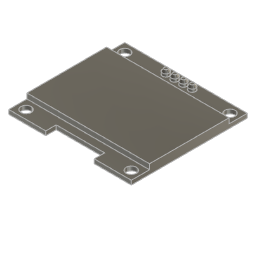
Reed Machine Case v17 (Autodesk Fusion 360 archive; units mm, degrees)
design "SSH1106+128x64+IIC+OLED+Display+1.3_+v3"
Autodesk Fusion 360 part; units mm, degrees
sketch "Sketch1" plane through (0, 0, 0) normal (0, 0, 1) x (1, 0, 0)
  line L0 (14.71, 7.35) -> (-14.71, 7.35)
  line L1 (-14.71, 7.35) -> (-14.71, -7.35)
  line L2 (-14.71, -7.35) -> (14.71, -7.35)
  line L3 (14.71, -7.35) -> (14.71, 7.35)
  line L4 (14.71, 7.35) -> (-14.71, -7.35) construction
  line L5 (-14.71, 7.35) -> (14.71, -7.35) construction
  line L6 (-17.7, 7.35) -> (-17.7, 14.7)
  line L7 (-17.7, 14.7) -> (-14.71, 14.7)
  line L8 (-17.7, 14.7) -> (17.7, 14.7)
  line L9 (17.7, 14.7) -> (17.7, -18.8)
  line L10 (17.7, -18.8) -> (-17.7, -18.8)
  line L11 (-17.7, -18.8) -> (-17.7, 14.7)
  line L12 (-17.7, 14.7) -> (6.5694, 14.7)
  line L13 (6.5694, 9.45) -> (-14.71, 9.45)
  line L14 (-17.7, 9.45) -> (-17.7, 14.7)
  line L15 (17.7, 9.45) -> (-17.7, 9.45)
  line L16 (-17.7, 9.45) -> (-17.7, -13.55)
  line L17 (-17.7, -13.55) -> (17.7, -13.55)
  line L18 (17.7, -13.55) -> (17.7, 9.45)
  line L19 (-17.7, 14.7) -> (-15.2, 14.7)
  line L20 (-15.2, 14.7) -> (-15.2, 12.2)
  line L21 (-15.2, 12.2) -> (-17.7, 12.2)
  line L22 (-17.7, 12.2) -> (-17.7, 14.7)
  circle A0 centre (-15.2, 12.2) radius 1.5
  circle A1 centre (15.2, 12.2) radius 1.5
  circle A2 centre (-15.2, -16.3) radius 1.5
  circle A3 centre (15.2, -16.3) radius 1.5
  line L23 (-17.7, -18.8) -> (-7, -18.8)
  line L24 (-7, -18.8) -> (-7, -17.6734)
  line L25 (-7, -17.6734) -> (-17.7, -17.6734)
  line L26 (-17.7, -17.6734) -> (-17.7, -18.8)
  line L27 (-7, -18.8) -> (7, -18.8)
  line L28 (7, -18.8) -> (7, -15.8)
  line L29 (7, -15.8) -> (-7, -15.8)
  line L30 (-7, -15.8) -> (-7, -18.8)
  line L31 (-17.7, 14.7) -> (-3.81, 14.7)
  line L32 (-3.81, 14.7) -> (-3.81, 12.7)
  line L33 (-3.81, 12.7) -> (-17.7, 12.7)
  line L34 (-17.7, 12.7) -> (-17.7, 14.7)
  circle A4 centre (-3.81, 12.7) radius 1
  circle A5 centre (-3.81, 12.7) radius 1
  circle A6 centre (-3.81, 12.7) radius 1
  circle A7 centre (-1.27, 12.7) radius 1
  circle A8 centre (1.27, 12.7) radius 1
  circle A9 centre (3.81, 12.7) radius 1
  circle A10 centre (-3.81, 12.7) radius 0.5
  circle A11 centre (-1.27, 12.7) radius 0.5
  circle A12 centre (1.27, 12.7) radius 0.5
  circle A13 centre (3.81, 12.7) radius 0.5
  line L35 (-2.81, 13.7) -> (-4.81, 13.7)
  line L36 (-4.81, 13.7) -> (-4.81, 11.7)
  line L37 (-4.81, 11.7) -> (-2.81, 11.7)
  line L38 (-2.81, 11.7) -> (-2.81, 13.7)
  line L39 (-2.81, 13.7) -> (-4.81, 11.7) construction
  line L40 (-4.81, 13.7) -> (-2.81, 11.7) construction
  line L41 (-0.27, 13.7) -> (-2.27, 13.7)
  line L42 (-2.27, 13.7) -> (-2.27, 11.7)
  line L43 (-2.27, 11.7) -> (-0.27, 11.7)
  line L44 (-0.27, 11.7) -> (-0.27, 13.7)
  line L45 (-0.27, 13.7) -> (-2.27, 11.7) construction
  line L46 (-2.27, 13.7) -> (-0.27, 11.7) construction
  line L47 (2.27, 13.7) -> (0.27, 13.7)
  line L48 (0.27, 13.7) -> (0.27, 11.7)
  line L49 (0.27, 11.7) -> (2.27, 11.7)
  line L50 (2.27, 11.7) -> (2.27, 13.7)
  line L51 (2.27, 13.7) -> (0.27, 11.7) construction
  line L52 (0.27, 13.7) -> (2.27, 11.7) construction
  line L53 (4.81, 13.7) -> (2.81, 13.7)
  line L54 (2.81, 13.7) -> (2.81, 11.7)
  line L55 (2.81, 11.7) -> (4.81, 11.7)
  line L56 (4.81, 11.7) -> (4.81, 13.7)
  line L57 (4.81, 13.7) -> (2.81, 11.7) construction
  line L58 (2.81, 13.7) -> (4.81, 11.7) construction
  point P0 (-3.81, 12.7)
  point P1 (-1.27, 12.7)
  point P2 (1.27, 12.7)
  point P3 (3.81, 12.7)
  dimension "d1" = 29.42
  dimension "d2" = 14.7
  dimension "d3" = 2.99
  dimension "d5" = 35.4
  dimension "d6" = 33.5
  dimension "d7" = 5.25
  dimension "d8" = 23
  dimension "d9" = 2.5
  dimension "d10" = 2.5
  dimension "d11" = 3
  dimension "d12" = 3
  dimension "d13" = 3
  dimension "d14" = 3
  dimension "d19" = 10.7
  dimension "d20" = 14
  dimension "d21" = 3
  dimension "d24" = 13.89
  dimension "d25" = 2
  dimension "d26" = 2
  dimension "d27" = 2
  dimension "d28" = 2
  dimension "d29" = 2
  dimension "d30" = 2
  dimension "d31" = 2
  dimension "d34" = 1
  dimension "d35" = 1
  dimension "d36" = 1
  dimension "d37" = 1
  dimension "d42" = 2
  dimension "d43" = 2
  dimension "d44" = 2
  dimension "d45" = 2
  dimension "d46" = 2
  dimension "d47" = 2
  dimension "d48" = 2
  dimension "d49" = 2
  constraint horizontal L0
  constraint perpendicular L0 L1
  constraint parallel L0 L2
  constraint parallel L1 L3
  constraint coincident L4 origin
  constraint coincident L5 origin
  constraint vertical L6
  constraint horizontal L7
  constraint horizontal L8
  constraint vertical L9
  constraint horizontal L10
  constraint vertical L11
  constraint horizontal L12
  constraint horizontal L13
  constraint vertical L14
  constraint horizontal L15
  constraint vertical L16
  constraint horizontal L17
  constraint vertical L18
  constraint coincident L9 L15.start
  constraint horizontal L19
  constraint vertical L20
  constraint horizontal L21
  constraint vertical L22
  constraint coincident L20.end L21.start
  constraint horizontal L23
  constraint vertical L24
  constraint horizontal L25
  constraint vertical L26
  constraint horizontal L27
  constraint vertical L28
  constraint horizontal L29
  constraint vertical L30
  constraint horizontal L31
  constraint vertical L32
  constraint horizontal L33
  constraint vertical L34
  constraint coincident P0 L32.end
  constraint concentric A5 A10
  constraint concentric A7 A11
  constraint concentric A8 A12
  constraint concentric A9 A13
  constraint horizontal L35
  constraint perpendicular L35 L36
  constraint parallel L35 L37
  constraint parallel L36 L38
  constraint coincident L39 P0
  constraint coincident L40 P0
  constraint horizontal L41
  constraint perpendicular L41 L42
  constraint parallel L41 L43
  constraint parallel L42 L44
  constraint coincident L45 P1
  constraint coincident L46 P1
  constraint coincident P1 A7.centre
  constraint horizontal L47
  constraint perpendicular L47 L48
  constraint parallel L47 L49
  constraint parallel L48 L50
  constraint coincident L51 P2
  constraint coincident L52 P2
  constraint coincident P2 A8.centre
  constraint horizontal L53
  constraint perpendicular L53 L54
  constraint parallel L53 L55
  constraint parallel L54 L56
  constraint coincident L57 P3
  constraint coincident L58 P3
  constraint coincident P3 A9.centre
  measures "d1" distance of L1.end L2.end
  measures "d2" distance of L0.end L1.end
  measures "d3" distance of L0.end L6.start
  measures "d5" distance of L6.end L8.end
  measures "d6" distance of L6.end L10.end
  measures "d7" distance of L6.end L14.start
  measures "d8" distance of L15.start L17.end
  measures "d9" distance of L6.end L19.end
  measures "d10" distance of L6.end L21.end
  measures "d11" diameter of A0
  measures "d12" diameter of A1
  measures "d13" diameter of A2
  measures "d14" diameter of A3
  measures "d19" distance of L10.end L23.end
  measures "d20" distance of L23.end L27.end
  measures "d21" distance of L23.end L29.end
  measures "d24" distance of L6.end L31.end
  measures "d25" distance of L6.end L33.end
  measures "d26" diameter of A4
  measures "d27" diameter of A5
  measures "d28" diameter of A6
  measures "d29" diameter of A7
  measures "d30" diameter of A8
  measures "d31" diameter of A9
  measures "d34" diameter of A10
  measures "d35" diameter of A11
  measures "d36" diameter of A12
  measures "d37" diameter of A13
  measures "d42" distance of L36.end L37.end
  measures "d43" distance of L35.end L36.end
  measures "d44" distance of L42.end L43.end
  measures "d45" distance of L41.end L42.end
  measures "d46" distance of L48.end L49.end
  measures "d47" distance of L47.end L48.end
  measures "d48" distance of L54.end L55.end
  measures "d49" distance of L53.end L54.end
extrude "Extrude1" add sketch "Sketch1" along normal blind 1.2 contours L0 L1 L2 L3 | L6 L9 L11 L13 L15 L16 L17 L18 | L6 L8 L9 L11 L12 L13 L14 L15 L21 A0 L32 L33 L35 L36 L37 L38 | L9 L10 L11 L17 A2 L25 L28 L29 L30 | L6 L11 L14 L21 L22 A0 L33 | L10 L11 A2 L23 L24 L25 L26 L30 | L6 L7 L8 L11 L12 L14 L19 L20 L22 A0 L31 L33 L34 | L10 L24 L27 L28 L29 L30 | L7 L8 L12 L20 A0 L31 L32 L33 L35 L36 | L32 L33 A4 A5 A6 A10 | A4 A5 A6 L35 L36 | L32 L33 A4 A5 A6 A10 | A4 A5 A6 L36 L37 | L32 L33 A10 | L32 L33 A10 | A4 A5 A6 L35 L38 | A4 A5 A6 L37 L38 | A7 | A7 L43 L44 | A7 L41 L44 | A7 L41 L42 | A7 L42 L43 | A8 | A8 L49 L50 | A8 L47 L50 | A8 L47 L48 | A8 L48 L49 | A9 | A9 L55 L56 | A9 L53 L56 | A9 L53 L54 | A9 L54 L55 | A11 | A12 | A13 makes body 1
extrude "Extrude2" add sketch "Sketch1" along normal blind 2.7 contours L0 L1 L2 L3 | L6 L9 L11 L13 L15 L16 L17 L18 bodies 1
extrude "Extrude3" cut sketch "Sketch1" along normal blind 1.2 contours L10 L24 L27 L28 L29 L30 bodies 1
extrude "Extrude4" add sketch "Sketch1" along normal blind 2 separate body contours L32 L33 A4 A5 A6 A10 | L32 L33 A4 A5 A6 A10 | L32 L33 A10 | L32 L33 A10 | A7 | A8 | A9 | A11 | A12 | A13 makes body 2 at (-0.2712, 12.6502, 0.6667) makes body 3 at (2.2688, 12.6502, 0.6667) makes body 4 at (-2.8112, 12.6502, 0.6667) makes body 5 at (4.805, 12.7996, 1.3333)
extrude "Extrude5" add sketch "Sketch1" along normal blind 2.7 contours L32 L33 A10 | L32 L33 A10 | A11 | A12 | A13 bodies 1 2 3 4 5
chamfer "Chamfer1" distance 0.7 distance2 0.5 4 edges at (3.3438, 12.5192, 2) (0.8038, 12.5192, 2) (-1.7362, 12.5192, 2) (-4.2762, 12.5192, 2) measured on face at (4.3075, 12.7498, 2.2333) measured on face at (1.7675, 12.7498, 2.2333) measured on face at (-0.7725, 12.7498, 2.2333) measured on face at (-3.3125, 12.7498, 2.4667) on bodies 1
extrude "Extrude6" add sketch "Sketch1" against normal blind 2 contours L32 L33 A4 A5 A6 A10 | A4 A5 A6 L35 L36 | L32 L33 A4 A5 A6 A10 | A4 A5 A6 L36 L37 | L32 L33 A10 | L32 L33 A10 | A4 A5 A6 L35 L38 | A4 A5 A6 L37 L38 | A7 | A7 L43 L44 | A7 L41 L44 | A7 L41 L42 | A7 L42 L43 | A8 | A8 L49 L50 | A8 L47 L50 | A8 L47 L48 | A8 L48 L49 | A9 | A9 L55 L56 | A9 L53 L56 | A9 L53 L54 | A9 L54 L55 | A11 | A12 | A13 bodies 1
extrude "Extrude7" add sketch "Sketch1" against normal blind 8.6 contours L32 L33 A10 | L32 L33 A10 | A11 | A12 | A13 bodies 1
fillet "Fillet1" radius 0.5 4 edges at (3.3438, 12.8808, -8.6) (0.8038, 12.8808, -8.6) (-1.7362, 12.8808, -8.6) (-4.2762, 12.8808, -8.6) on bodies 1
